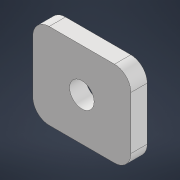
# Autodesk Inventor part: mount_linear_stepper_washer_c
Saved by Autodesk Inventor 2021 (Build 250183000, 183)
## iProperties
Created: 2020-12-29
Part Number: mount_linear_stepper_washer_c
Material: Generic
Document SubType Name: Modeling
Designer: Tomasz
Density: 1 g/cm^3
Appearance: Default
Author: Tomasz
Autodesk Inventor part; units mm, degrees
ref_plane "YZ Plane" through (0, 0, 0) normal (1, 0, 0) x (0, 1, 0)
ref_plane "XZ Plane" through (0, 0, 0) normal (0, 1, 0) x (-1, 0, 0)
ref_plane "XY Plane" through (0, 0, 0) normal (0, 0, 1) x (1, 0, 0)
sketch "washer_sketch" plane through (0, 0, 0) normal (0, 0, 1) x (1, 0, 0)
  line L0 (4.6466, -2.6825) -> (1.9799, -4.6825) construction
  arc A0 (4.6466, -2.6825) -> (5.4466, -1.0825) centre (3.4466, -1.0825) ccw construction
  line L1 (5.4466, 5.0715) -> (5.4466, -1.0825) construction
  line L2 (5.4466, 5.0825) -> (5.4466, 5.0715) construction
  line L3 (-5.4466, 5.0825) -> (5.4466, 5.0825) construction
  line L4 (-5.4466, 0.6191) -> (-5.4466, 5.0825) construction
  arc A1 (-5.4466, 0.6191) -> (-5.0083, -0.6303) centre (-3.4466, 0.6191) ccw construction
  line L5 (-2.0471, -4.3319) -> (-5.0083, -0.6303) construction
  arc A2 (-2.0471, -4.3319) -> (-0.4853, -5.0825) centre (-0.4853, -3.0825) ccw construction
  line L6 (0.7799, -5.0825) -> (-0.4853, -5.0825) construction
  arc A3 (0.7799, -5.0825) -> (1.9799, -4.6825) centre (0.7799, -3.0825) ccw construction
  circle A4 centre (0.0413, -0.1642) radius 3.55 construction
  circle A5 centre (0.0413, -0.1642) radius 3.55 construction
  circle A6 centre (0.0413, -0.1642) radius 1.5 projected
  line L7 (-3.9587, -5.4) -> (4.0413, -5.4)
  line L8 (6.0413, -3.4) -> (6.0413, 3.0715)
  line L9 (4.0413, 5.0715) -> (-3.9587, 5.0715)
  line L10 (-5.9587, 3.0715) -> (-5.9587, -3.4)
  arc A7 (-5.9587, -3.4) -> (-3.9587, -5.4) centre (-3.9587, -3.4) ccw
  arc A8 (-3.9587, 5.0715) -> (-5.9587, 3.0715) centre (-3.9587, 3.0715) ccw
  arc A9 (6.0413, 3.0715) -> (4.0413, 5.0715) centre (4.0413, 3.0715) ccw
  arc A10 (4.0413, -5.4) -> (6.0413, -3.4) centre (4.0413, -3.4) ccw
  point P0 (0, 0)
  point P1 (-5.9587, -5.4)
  point P2 (6.0413, 5.0715)
  point P3 (6.0413, -5.4)
  point P4 (-5.9587, 5.0715)
  dimension "d0" = 10.4715
  dimension "d1" = 12
  dimension "d2" = 5.2358
  dimension "d3" = 6
  dimension "d4" = 2
  constraints: 8 end point, 8 point on circle, 8 point on line, 8 tangent, 4 centre point, 3 equal radius, 2 parallel, 1 horizontal, 1 horizontal alignment, 1 perpendicular
  measures "d0" distance of point (-5.959, 5.072) point (-5.959, -5.4)
  measures "d1" distance of point (-5.959, -5.4) point (6.041, -5.4)
  measures "d2" distance from line of L9 A6.centre
  measures "d3" distance from line of A4.centre L10
  measures "d4" radius of A7
extrude "washer" add sketch "washer_sketch" along normal blind 2
equation "\"d0\" = 2 * d2"
equation "\"d3\" = 0.5 * d1"
body "Solid1"
